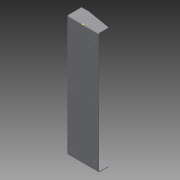
# Autodesk Inventor part: obodowka_cz_2
Saved by Autodesk Inventor 2015 (Build 190159000, 159)
## iProperties
Created: 2015-09-19
Part Number: obodowka_cz_2
Material: Generic
Document SubType Name: Sheet Metal
Designer: Komp
Density: 1 g/cm^3
Flat Pattern Width: 7.7 cm
Flat Pattern Length: 36.4786 cm
Flat Pattern Area: 280.885 cm^2
Sheet Metal Rule: Default_mm
Sheet Metal Width: 77,000 mm
Sheet Metal Length: 364,786 mm
Sheet Metal Area: 28088,510 mm^2
Appearance: Default
Author: Komp
Autodesk Inventor part; units mm, degrees
ref_plane "YZ Plane" through (0, 0, 0) normal (1, 0, 0) x (0, 1, 0)
ref_plane "XZ Plane" through (0, 0, 0) normal (0, 1, 0) x (-1, 0, 0)
ref_plane "XY Plane" through (0, 0, 0) normal (0, 0, 1) x (1, 0, 0)
sketch "Sketch1" plane through (0, 0, 0) normal (0, 1, 0) x (-1, 0, 0)
  line L0 (38.5, 73.5) -> (-38.5, 73.5)
  line L1 (-38.5, 73.5) -> (-38.5, -73.5)
  line L2 (-38.5, -73.5) -> (38.5, -73.5)
  line L3 (38.5, -73.5) -> (38.5, 73.5)
  line L4 (38.5, 73.5) -> (-38.5, -73.5) construction
  line L5 (-38.5, 73.5) -> (38.5, -73.5) construction
  point P0 (0, 0)
  dimension "d0" = 77
  dimension "d1" = 147
  measures "d0" distance of L1.end L2.end
  measures "d1" distance of L0.end L1.end
extrude "Plate1" add sketch "Sketch1" along normal blind 1.5
sketch "Sketch2" plane through (38.5, 3, 75) normal (0, 0, 1) x (1, 0, 0)
  line L0 (-77, 0) -> (0, 0)
  line L1 (0, 0) -> (0, 32)
  line L2 (0, 32) -> (-77, 32)
  line L3 (-77, 32) -> (-77, 0)
  constraints: 6 end point, 1 horizontal, 1 perpendicular, 1 vertical
edge flange "Flange1" height 35 angle 90 thickness 1.5 bend radius 1.5 thickness toward (0, 0, 1) relief straight relief width 1.5 relief depth 0.75 edges at (0, 1.5, 73.5) wall of the first edge with corners at (-38.5, 3, 75) (38.5, 3, 75) (38.5, 35, 75) (-38.5, 35, 75)
bend "Bend1"
corner "Corner1"
chamfer "Corner Chamfer1" distance 10 distance2 58.5 1 edges at (38.5, 35, 75.75) measured on face at (38.5, 34.5, 75.75)
fillet "Corner Round1" radius 0.25 1 edges at (38.5, 25, 75.75)
fillet "Corner Round2" radius 0.25 1 edges at (-38.5, 35, 75.75)
mirror "Mirror1" about plane through (-38.5, 0, -73.5) normal (0, 0, -1) of "Flange1", "Plate1"
chamfer "Corner Chamfer2" distance 58.5 distance2 10 1 edges at (38.5, 35, -222.75) measured on face at (38, 35, -222.75)
fillet "Corner Round3" radius 0.25 1 edges at (38.5, 25, -222.75)
fillet "Corner Round5" radius 0.25 1 edges at (-38.5, 35, -222.75)
hole "Hole1" at (28, 0, 56.5) direction (0, 1, 0) diameter 3.2 depth 1.5 tip angle 118
hole "Hole2" at (-28, 0, 56.5) direction (0, 1, 0) diameter 3.2 depth 1.5 tip angle 118
hole "Hole3" at (28, 0, -203.5) direction (0, 1, 0) diameter 3.2 depth 1.5 tip angle 118
hole "Hole4" at (-28, 0, -203.5) direction (0, 1, 0) diameter 3.2 depth 1.5 tip angle 118
hole "Hole5" at (28, 0, -73.5) direction (0, 1, 0) diameter 3.2 depth 1.5 tip angle 118
hole "Hole6" at (-28, 0, -73.5) direction (0, 1, 0) diameter 3.2 depth 1.5 tip angle 118
sketch "Sketch3" plane through (0, 1.5, 0) normal (0, 1, 0) x (1, 0, 0)
  point P0 (0, 0)
sketch "Sketch4" plane through (-38.5, 3, 76.5) normal (0, 0, 1) x (1, 0, 0)
  point P0 (38.5, -3)
equation "\"d31\" = Thickness"
equation "\"d40\" = Thickness"
equation "\"d49\" = Thickness"
equation "\"d58\" = Thickness"
equation "\"d67\" = Thickness"
equation "\"d76\" = Thickness"
equation "\"d3\" = BendReliefWidth"
equation "\"d4\" = BendReliefDepth"
equation "\"d5\" = MinimumRemnant"
equation "\"d6\" = BendRadius"
equation "\"d9\" = BendRadius"
equation "\"d10\" = CornerReliefSize"
equation "\"d11\" = GapSize"
equation "\"d12\" = JacobiRadiusSize"
equation "\"BendRadius\" = Thickness"
equation "\"BendReliefWidth\" = Thickness"
equation "\"BendReliefDepth\" = 0.5 * Thickness"
equation "\"CornerReliefSize\" = 4 * Thickness"
equation "\"MinimumRemnant\" = 2 * Thickness"
equation "\"TransitionRadius\" = BendRadius"
equation "\"JacobiRadiusSize\" = BendRadius"
equation "\"GapSize\" = Thickness"
equation "\"d2\" = BendRadius"
equation "\"Thickness\" = 1.5"
body "Solid1"
